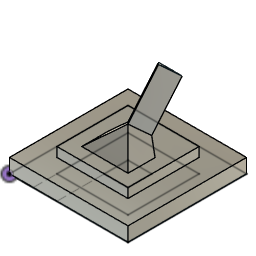
l02_wall_hook (Autodesk Fusion 360 design; units mm, degrees)
part number: 2025-08-21-18-47-32-651
Autodesk Fusion 360 part; units mm, degrees
sketch "Sketch1" plane through (0, 0, 0) normal (0, 0, 1) x (1, 0, 0)
  line L0 (0, 0) -> (25, 0)
  line L1 (25, 0) -> (25, 25)
  line L2 (25, 25) -> (0, 25)
  line L3 (0, 25) -> (0, 0)
  line L4 (0, 0) -> (10, 0) construction
  line L5 (10, 0) -> (10, 10) construction
  line L6 (10, 10) -> (15, 10)
  line L7 (15, 10) -> (15, 15)
  line L8 (15, 15) -> (10, 15)
  line L9 (10, 15) -> (10, 10)
  line L10 (0, 0) -> (5, 0) construction
  line L11 (0, 0) -> (5, 0) construction
  line L12 (5, 0) -> (5, 5) construction
  line L13 (5, 5) -> (20, 5)
  line L14 (20, 5) -> (20, 20)
  line L15 (20, 20) -> (5, 20)
  line L16 (5, 20) -> (5, 5)
  dimension "d1" = 25
  dimension "d2" = 25
  dimension "d3" = 10
  dimension "d4" = 10
  dimension "d5" = 5
  dimension "d6" = 5
  dimension "d7" = 5
  dimension "d8" = 5
  dimension "d9" = 15
  dimension "d10" = 15
  constraint horizontal L0
  constraint vertical L1
  constraint horizontal L2
  constraint vertical L3
  constraint coincident L0.start L3.end
  constraint perpendicular L3 L4
  constraint perpendicular L0 L5
  constraint horizontal L6
  constraint vertical L7
  constraint horizontal L8
  constraint vertical L9
  constraint midpoint L4 L10.end
  constraint parallel L4 L11
  constraint perpendicular L11 L12
  constraint horizontal L13
  constraint vertical L14
  constraint horizontal L15
  constraint vertical L16
  measures "d1" distance of L0.start L0.end
  measures "d2" distance of L0.start L2.end
  measures "d3" distance of L0.start L4.end
  measures "d4" distance of L4.end L5.end
  measures "d5" distance of L5.end L6.end
  measures "d6" distance of L5.end L8.end
  measures "d7" distance of L0.start L10.end
  measures "d8" distance of L10.end L12.end
  measures "d9" distance of L12.end L13.end
  measures "d10" distance of L12.end L15.end
extrude "Extrude1" add sketch "Sketch1" along normal blind 3 contours L0 L1 L2 L3 | L6 L7 L8 L9 | L13 L14 L15 L16
extrude "Extrude2" cut 1 faces at (8.3333, 16.6667, 3) along direction (0, 0, -1) blind 3
extrude "Extrude3" add sketch "Sketch1" along normal blind 3 contours L0 L1 L2 L3
extrude "Extrude4" add sketch "Sketch1" along normal blind 5 contours L13 L14 L15 L16
extrude "Extrude5" add sketch "Sketch1" along normal blind 7 contours L6 L7 L8 L9
extrude "Extrude6" add 1 faces at (13.3333, 11.6667, 7) along direction (0, 0, 1) blind 10 draft -50
extrude "Extrude7" add 1 faces at (12.5, 14.1667, 7.6993) along direction (0, 0.642788, 0.766044) blind 10
delete_face "DeleteFace1" 1 faces at (15, 11.6667, 5.6667)
delete_face "DeleteFace2" 1 faces at (14.1278, 10, 5.6667)
delete_face "DeleteFace3" 1 faces at (10, 10.8722, 5.6667)
delete_face "DeleteFace4" 1 faces at (13.3333, 15, 5.6667)
sketch "Sketch2" plane through (0, 16.0723, 19.1543) normal (0, 0.642788, 0.766044) x (-1, 0, 0)
  line L0 (-10, -6.9912) -> (-12.5, -3.7276)
  line L1 (-12.5, -3.7276) -> (-15, -6.9912)
  line L2 (-15, -6.9912) -> (-10, -6.9912)
